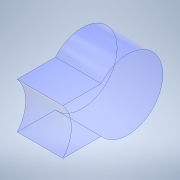
# Autodesk Inventor part: knee
Saved by Autodesk Inventor 2020.2 (Build 242310000, 310)
## iProperties
Created: 2021-01-30
Part Number: knee
Material: Generic
Document SubType Name: Modeling
Designer: DELL
Density: 1 g/cm^3
Appearance: Clear - Blue
Author: DELL
Autodesk Inventor part; units mm, degrees
ref_plane "YZ Plane" through (0, 0, 0) normal (1, 0, 0) x (0, 1, 0)
ref_plane "XZ Plane" through (0, 0, 0) normal (0, 1, 0) x (-1, 0, 0)
ref_plane "XY Plane" through (0, 0, 0) normal (0, 0, 1) x (1, 0, 0)
sketch "Sketch17" plane through (0, 0, 0) normal (1, 0, 0) x (0, 1, 0)
  line L0 (-64.4, 0) -> (64.4, 0) construction
  line L1 (0, -208.4) -> (0, 88.4) projected
  circle A0 centre (0, 0) radius 40
  circle A1 centre (0, 0) radius 46
  line L2 (-30, -34.8712) -> (-30, -85.1288)
  line L3 (30, -85.1288) -> (30, -34.8712)
  circle A2 centre (0, -120) radius 46
  circle A3 centre (0, -120) radius 40
  point P0 (0, -46)
  point P1 (0, 46)
  dimension "d173" = 92
  dimension "d174" = 80
  dimension "d246" = 60
  dimension "d247" = 80
  dimension "d248" = 92
  dimension "d249" = 120
  dimension "d253" = 50.2576
  constraints: 4 centre point, 4 end point, 4 point on circle, 3 coincident, 1 point on line, 1 vertical, 1 other
  measures "d173" diameter of A1
  measures "d174" diameter of A0
  measures "d246" distance between parallel lines of L3 L2
  measures "d247" diameter of A3
  measures "d248" diameter of A2
  measures "d249" distance of A2.centre point (0, 0)
  measures "d253" distance of L3.start L3.end
extrude "Extrusion18" add sketch "Sketch17" along normal mid plane 60 contours A2 L1 A3 | L1 A3 A2 | A3 L1 | L1 A3 | L2 A1 L1 A2 | L1 A1 L3 A2
fillet "Fillet17" [suppressed]
body "Solid1"
body "Solid9"
